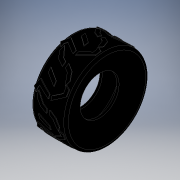
# Autodesk Inventor part: RCT-P010 Wheel
Saved by Autodesk Inventor 2019 (Build 230136000, 136)
## iProperties
Created: 2019-10-03
Part Number: RCT-P010 Wheel
Material: Genérico
Document SubType Name: Modeling
Designer: david
Density: 1 g/cm^3
Appearance: Valor por defecto
Author: david
Autodesk Inventor part; units mm, degrees
ref_plane "YZ Plane" through (0, 0, 0) normal (1, 0, 0) x (0, 1, 0)
ref_plane "XZ Plane" through (0, 0, 0) normal (0, 1, 0) x (-1, 0, 0)
sketch "Boceto1" plane through (0, 0, 0) normal (0, 0, 1) x (1, 0, 0)
  line L0 (0, 0) -> (3.0911, 0)
  line L1 (3.0911, 0) -> (0, 0) construction
  line L2 (0, 0) -> (0, 28.54) construction
  line L3 (0, 60.74) -> (53.1, 60.74)
  line L4 (26.55, 28.54) -> (37.2, 28.54) construction
  line L5 (26.55, 28.54) -> (15.9, 28.54) construction
  line L6 (26.55, 28.54) -> (37.2, 28.54) construction
  line L7 (15.9, 28.54) -> (12.4, 28.54)
  line L8 (37.2, 28.54) -> (40.7, 28.54)
  line L9 (40.7, 28.54) -> (53.1, 60.74)
  line L10 (23.0246, 60.74) -> (28.5246, 60.74) construction
  line L11 (37.2, 55.24) -> (37.2, 28.54)
  line L12 (0, 60.74) -> (12.4, 28.54)
  line L13 (15.9, 28.54) -> (15.9, 55.24)
  line L14 (37.2, 55.24) -> (15.9, 55.24)
  dimension "d18" = 0
  dimension "d0" = 28.54
  dimension "d4" = 26.55
  dimension "d5" = 10.65
  dimension "d6" = 10.65
  dimension "d7" = 180
  dimension "d8" = 3.5
  dimension "d9" = 3.5
  dimension "d12" = 21.3
  dimension "d13" = 53.1
  dimension "d14" = 32.2
  dimension "d15" = 32.2
  dimension "d17" = 26.7
  constraints: 30 end point, 9 horizontal, 5 point on line, 2 collinear, 2 vertical, 10 other
  measures "d0" distance of L0.start L2.end
  measures "d4" distance of L2.end L4.start
  measures "d5" distance of L4.start L4.end
  measures "d6" distance of L4.start L5.end
  measures "d7" angle of L5 L6
  measures "d8" distance of L5.end L7.end
  measures "d9" distance of L6.end L8.end
  measures "d12" distance of L11.start L13.end
  measures "d13" distance of point (0, 60.74) point (53.1, 60.74)
  measures "d14" vertical distance of L8.end point (53.1, 60.74)
  measures "d15" vertical distance of point (0, 60.74) L7.end
  measures "d17" distance of L11.start L6.end
revolve "Revolución1" add sketch "Boceto1" angle 360 about axis through (0, 0, 0) along (1, 0, 0)
ref_plane "Plano de trabajo2" through (26.55, 0, 60.74) normal (0, 0, 1) x (1, 0, 0)
ref_plane "Plano de trabajo1" through (26.55, 0, 60.74) normal (0, 0, 1) x (1, 0, 0)
sketch "Boceto2" plane through (26.55, 0, 60.74) normal (0, 0, 1) x (1, 0, 0)
  line L0 (-26.55, 0) -> (26.55, 0) construction
  line L1 (26.55, -60.74) -> (26.55, 60.74) construction
  line L2 (-26.55, 60.74) -> (26.55, 60.74) construction
  line L3 (0, 60.74) -> (0, 0) construction
  line L4 (-26.55, -60.74) -> (26.55, -60.74) construction
  line L5 (0, -60.74) -> (0, 0) construction
  line L6 (26.55, 0) -> (26.55, -60.74) construction
  line L7 (26.55, -60.74) -> (26.55, 60.74) construction
  line L8 (26.55, 60.74) -> (-26.55, 60.74) construction
  line L9 (-26.55, 60.74) -> (-26.55, -60.74) construction
  line L10 (-2.2965, 0) -> (-11.1325, 4.6824)
  line L11 (-11.1325, 4.6824) -> (-17.0966, 12.7092)
  line L12 (-7.5472, 8.6366) -> (-13.2743, 15.9325)
  line L13 (-2.2965, 0) -> (-2.2965, 5.9568)
  line L14 (-17.0966, 12.7092) -> (-17.0966, 20.4652)
  line L15 (-17.0966, 20.4652) -> (-13.2743, 15.9325)
  line L16 (-2.2965, 5.9568) -> (-7.5472, 8.6366)
  line L17 (0, -60.74) -> (0, 0) construction
  line L18 (2.2965, 0.189) -> (7.5472, -3.0073)
  line L19 (13.2743, -15.655) -> (7.5472, -3.0073)
  line L20 (15.8962, -9.3311) -> (11.463, 0.459)
  line L21 (11.463, 0.459) -> (4.8948, 4.4574)
  line L22 (2.2965, 0.189) -> (2.2965, 6.0391)
  line L23 (2.2965, 6.0391) -> (4.8948, 4.4574)
  line L24 (13.2743, -15.655) -> (15.8962, -9.3311)
  line L25 (-19.4818, 17.2543) -> (-19.4818, 21.7019)
  line L26 (-19.4818, 21.7019) -> (-17.4618, 25.5138)
  line L27 (-17.4618, 25.5138) -> (-1.8835, 17.2586)
  line L28 (-19.5344, 31.4802) -> (-24.4718, 22.1631)
  line L29 (-19.4818, 17.2543) -> (-24.4718, 22.1631)
  line L30 (-1.8835, 17.2586) -> (-1.8835, 22.1266)
  line L31 (0.04, 20.8884) -> (0, 20.9096)
  line L32 (-1.8835, 22.1266) -> (-19.5344, 31.4802)
  line L33 (1.8835, 17.2586) -> (1.8835, 22.1266)
  line L34 (15.0606, 29.8887) -> (1.8835, 22.1266)
  line L35 (15.0606, 29.8887) -> (15.0606, 33.7006)
  line L36 (15.0606, 33.7006) -> (12.9815, 37.6242)
  line L37 (19.9606, 28.3237) -> (1.8835, 17.2586)
  line L38 (12.9815, 37.6242) -> (19.9606, 35.0563)
  line L39 (19.9606, 28.3237) -> (19.9606, 35.0563)
  dimension "d20" = 10
  dimension "d21" = 10
  dimension "d24" = 2.2965
  dimension "d28" = 5.2507
  dimension "d29" = 5.2507
  dimension "d30" = 5.7271
  dimension "d31" = 3.8223
  dimension "d34" = 5.7271
  dimension "d36" = 4.997
  dimension "d39" = 10.5445
  dimension "d40" = 3.8119
  dimension "d41" = 3.8119
  dimension "d42" = 152.08
  dimension "d43" = 152.08
  constraints: 74 end point, 8 vertical, 6 perpendicular, 4 midpoint, 3 point on line, 2 symmetric about line
  measures "d20" distance of L10.start L10.end
  measures "d21" distance of L10.end L11.end
  measures "d24" distance between parallel lines of L3 L13
  measures "d28" horizontal distance of L13.end L12.start
  measures "d29" horizontal distance of L18.start L18.end
  measures "d30" horizontal distance of L12.start L12.end
  measures "d31" horizontal distance of L14.end L12.end
  measures "d34" horizontal distance of L18.end L19.start
  measures "d36" distance between parallel lines of L19 L20
  measures "d39" distance of L28.start L28.end
  measures "d40" vertical distance of L25.end L26.end
  measures "d41" distance of L34.start L35.end
  measures "d42" angle of L25 L26
  measures "d43" angle of L35 L36
emboss "Repujado1" sketch "Boceto2" operation add depth 1 direction (0, 0, -1)
pattern_circular "Patrón circular1" count 7 over 360 about axis through (14.15, 0, 0) along (1, 0, 0) of "Repujado1"
sketch "Boceto3" plane through (26.55, 0, 60.74) normal (0, 0, 1) x (1, 0, 0)
  line L0 (-14.15, -28.54) -> (-14.15, 28.54) projected
  line L1 (-14.15, -6.4128) -> (-0.0046, -16.0949)
  line L2 (-0.0046, -16.0949) -> (-0.0046, -22.0655)
  line L3 (-0.0046, -22.0655) -> (-13.3084, -12.9595)
  line L4 (-13.3084, -12.9595) -> (-14.15, -6.4128)
  point P0 (-26.55, 0)
  constraints: 8 end point, 2 parallel, 1 point on line
emboss "Repujado2" sketch "Boceto3" operation add depth 1 direction (0, 0, -1)
pattern_circular "Patrón circular2" count 7 over 360 about axis through (38.95, 0, 0) along (1, 0, 0) of "Repujado2"
sketch "Boceto5" plane through (15.9, 0, 0) normal (1, 0, 0) x (0, 0, -1)
  point P0 (0, 0)
fillet "Empalme1" radius 3 2 edges at (0, -60.74, 0) (53.1, -60.74, 0)
equation "\"d9\" = d8"
equation "\"d17\" = d16"
equation "\"d29\" = d28"
equation "\"d41\" = d40"
equation "\"d43\" = d42"
equation "\"d15\" = d14"
equation "\"d16\" = 26.7"
